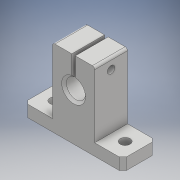
# Autodesk Inventor part: SH8
Saved by Autodesk Inventor 2018 (Build 220112000, 112)
## iProperties
Created: 2017-12-25
Part Number: SH8
Material: Generic
Document SubType Name: Modeling
Designer: Jurjen
Density: 1 g/cm^3
Appearance: Default
Author: Jurjen
Autodesk Inventor part; units mm, degrees
ref_plane "YZ Plane" through (0, 0, 0) normal (1, 0, 0) x (0, 1, 0)
ref_plane "XZ Plane" through (0, 0, 0) normal (0, 1, 0) x (-1, 0, 0)
ref_plane "XY Plane" through (0, 0, 0) normal (0, 0, 1) x (1, 0, 0)
sketch "Sketch1" plane through (0, 0, 0) normal (0, 1, 0) x (-1, 0, 0)
  line L0 (-21, -11.5) -> (-21, -16.5)
  line L1 (-21, -16.5) -> (0, -16.5)
  line L2 (0, -16.5) -> (0, 16.5) construction
  line L3 (0, 16.5) -> (-9, 16.5)
  line L4 (-9, 16.5) -> (-9, -11.5)
  line L5 (-9, -11.5) -> (-21, -11.5)
  line L6 (21, -11.5) -> (21, -16.5)
  line L7 (21, -16.5) -> (0, -16.5)
  line L8 (0, 16.5) -> (9, 16.5)
  line L9 (9, 16.5) -> (9, -11.5)
  line L10 (9, -11.5) -> (21, -11.5)
  point P0 (0, 0)
  point P1 (0, 0)
  dimension "d0" = 5
  dimension "d1" = 33
  dimension "d2" = 21
  dimension "d3" = 9
  constraints: 22 end point, 5 perpendicular, 4 symmetric about line, 1 coincident, 1 midpoint, 1 vertical, 1 vertical alignment
  measures "d0" distance between parallel lines of L1 L5
  measures "d1" distance between parallel lines of L3 L1
  measures "d2" distance between parallel lines of L2 L0
  measures "d3" distance between parallel lines of L2 L4
extrude "Extrusion1" add sketch "Sketch1" along normal mid plane 14
sketch "Sketch2" plane through (0, 7, 0) normal (0, 1, 0) x (1, 0, 0)
  arc A0 (0.75, -7.5054) -> (-0.75, -7.5054) centre (0, -3.5) ccw
  line L0 (-0.75, -16.5) -> (0.75, -16.5)
  line L1 (0.75, -16.5) -> (0.75, -7.5054)
  line L2 (-0.75, -7.5054) -> (-0.75, -16.5)
  line L3 (-9, -16.5) -> (9, -16.5) projected
  point P0 (0, 0)
  point P1 (0, -16.5)
  dimension "d6" = 8.15
  dimension "d7" = 13
  dimension "d8" = 1.5
  constraints: 6 end point, 2 point on circle, 2 vertical alignment, 1 centre point, 1 horizontal, 1 horizontal alignment, 1 midpoint, 1 parallel, 1 perpendicular
  measures "d6" diameter of A0
  measures "d7" distance from line of L3 A0.centre
  measures "d8" distance between parallel lines of L1 L2
extrude "Extrusion2" cut sketch "Sketch2" against normal through all
sketch "Sketch3" plane through (9, -7, -11.5) normal (1, 0, 0) x (0, 0, -1)
  circle A0 centre (-23.5, 7) radius 1.6
  line L0 (-28, 0) -> (-28, 14) projected
  point P0 (-11.5, 7)
  dimension "d11" = 3.2
  dimension "d13" = 4.5
  constraints: 1 centre point, 1 horizontal alignment
  measures "d11" diameter of A0
  measures "d13" distance from line of A0.centre L0
extrude "Extrusion3" cut sketch "Sketch3" against normal through all
sketch "Sketch4" plane through (-9, -7, 16.5) normal (-1, 0, 0) x (0, 0, 1)
  circle A0 centre (-4.5, 7) radius 1.6 projected
  line L0 (-6.1373, 4.15) -> (-2.8627, 4.15)
  line L1 (-2.8627, 4.15) -> (-1.25, 7)
  line L2 (-1.25, 7) -> (-2.8627, 9.85)
  line L3 (-2.8627, 9.85) -> (-6.1373, 9.85)
  line L4 (-6.1373, 9.85) -> (-7.75, 7)
  line L5 (-7.75, 7) -> (-6.1373, 4.15)
  point P0 (-16.5, 7)
  point P1 (-4.5, 4.15)
  point P2 (-4.5, 9.85)
  dimension "d16" = 5.7
  dimension "d17" = 6.5
  constraints: 12 end point, 3 parallel, 2 equal length, 2 horizontal alignment, 2 midpoint, 2 vertical alignment, 1 horizontal
  measures "d16" distance between parallel lines of L3 L0
  measures "d17" distance of L1.end L4.end
extrude "Extrusion4" cut sketch "Sketch4" against normal blind 2.6
sketch "Sketch5" plane through (-21, 7, -11.5) normal (0, 0, 1) x (1, 0, 0)
  circle A0 centre (6, -7) radius 2.1
  circle A1 centre (36, -7) radius 2.1
  line L0 (0, -14) -> (0, 0) projected
  line L1 (0, 0) -> (12, 0) projected
  line L2 (30, 0) -> (42, 0) projected
  point P0 (21, -7)
  point P1 (0, -7)
  point P2 (6, 0)
  point P3 (36, 0)
  dimension "d20" = 4.2
  constraints: 3 midpoint, 2 centre point, 2 horizontal alignment, 2 vertical alignment, 1 equal radius
  measures "d20" diameter of A0
extrude "Extrusion5" cut sketch "Sketch5" against normal through all
chamfer "Chamfer2" distance 1.5 angle 45 4 edges at (-21, 7, -14) (-21, -7, -14) (21, 7, -14) (21, -7, -14)
fillet "Fillet1" radius 1 2 edges at (-9, 0, 16.5) (9, 0, 16.5)
chamfer "Chamfer3" distance 1 angle 45 2 edges at (0, -7, -0.575) (0, 7, -0.575)
body "Solid1"
